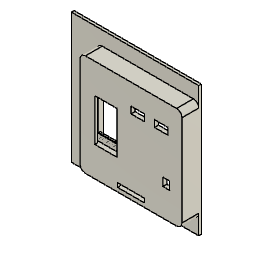
electronics_holder (Autodesk Fusion 360 design; units mm, degrees)
Autodesk Fusion 360 part; units mm, degrees
note: some values were not read from the file. Set by a fixed rule: which sketch regions a step uses.
sketch "Sketch1" plane through (0, 0, 0) normal (0, 1, 0) x (1, 0, 0)
  line L0 (0, 0) -> (190, 0)
  line L1 (190, 0) -> (190, -194)
  line L2 (190, -194) -> (0, -194)
  line L3 (0, -194) -> (0, 0)
  dimension "d1" = 190
  dimension "d2" = 194
  constraint horizontal L0
  constraint vertical L1
  constraint horizontal L2
  constraint vertical L3
  constraint coincident L0.start L3.end
  measures "d1" distance of L0.start L0.end
  measures "d2" distance of L0.end L1.end
extrude "Extrude1" add sketch "Sketch1" against normal blind 4
sketch "Sketch2" plane through (0, -4, 0) normal (0, -1, 0) x (1, 0, 0)
  line L0 (190, 194) -> (0, 194)
  line L1 (0, 194) -> (0, 0)
  line L2 (0, 0) -> (190, 0)
  line L3 (190, 0) -> (190, 194)
  line L4 (44, 167) -> (184, 167)
  line L5 (184, 167) -> (184, 27)
  line L6 (184, 27) -> (44, 27)
  line L7 (44, 27) -> (44, 167)
  dimension "d5" = 44
  dimension "d6" = 140
  dimension "d7" = 27
  dimension "d8" = 140
  constraint horizontal L4
  constraint vertical L5
  constraint horizontal L6
  constraint vertical L7
  measures "d5" distance of L1 L7
  measures "d6" distance of L5.end L6.end
  measures "d7" distance of L2 L6
  measures "d8" distance of L4.end L5.end
extrude "Extrude2" cut sketch "Sketch2" against normal blind 4 contours L4 L5 L6 L7
fillet "Fillet1" radius 8 4 edges at (44, -2, 167) (44, -2, 27) (184, -2, 167) (184, -2, 27)
sketch "Sketch3" plane through (0, -4, 0) normal (0, -1, 0) x (1, 0, 0)
  line L0 (184, 159) -> (184, 35)
  arc A0 (176, 27) -> (184, 35) centre (176, 35) ccw
  line L1 (176, 27) -> (52, 27)
  arc A1 (44, 35) -> (52, 27) centre (52, 35) ccw
  line L2 (44, 35) -> (44, 159)
  arc A2 (52, 167) -> (44, 159) centre (52, 159) ccw
  line L3 (52, 167) -> (176, 167)
  arc A3 (184, 159) -> (176, 167) centre (176, 159) ccw
  line L4 (190, 194) -> (0, 194)
  line L5 (0, 194) -> (0, 0)
  line L6 (0, 0) -> (190, 0)
  line L7 (190, 0) -> (190, 194)
  line L8 (38, 173) -> (190, 173)
  line L9 (190, 173) -> (190, 21)
  line L10 (190, 21) -> (38, 21)
  line L11 (38, 21) -> (38, 173)
  dimension "d13" = 6
  dimension "d14" = 6
  dimension "d15" = 6
  dimension "d16" = 6
  constraint horizontal L8
  constraint vertical L9
  constraint horizontal L10
  constraint vertical L11
  constraint coincident L7 L9.end
  measures "d13" distance of L0 L9
  measures "d14" distance of L2 L11
  measures "d15" distance of L1 L10
  measures "d16" distance of L3 L8
extrude "Extrude3" add sketch "Sketch3" along normal blind 21 contours L7 L8 L9 L10 L11
sketch "Sketch4" plane through (0, -25, 0) normal (0, -1, 0) x (1, 0, 0)
  arc A0 (176, 27) -> (184, 35) centre (176, 35) ccw
  line L0 (176, 27) -> (52, 27)
  arc A1 (44, 35) -> (52, 27) centre (52, 35) ccw
  line L1 (44, 35) -> (44, 159)
  arc A2 (52, 167) -> (44, 159) centre (52, 159) ccw
  line L2 (52, 167) -> (176, 167)
  arc A3 (184, 159) -> (176, 167) centre (176, 159) ccw
  line L3 (184, 159) -> (184, 35)
  line L4 (38, 21) -> (190, 21)
  line L5 (190, 21) -> (190, 173)
  line L6 (190, 173) -> (38, 173)
  line L7 (38, 173) -> (38, 21)
  line L8 (38, 173) -> (190, 173)
  line L9 (190, 173) -> (190, 21)
  line L10 (190, 21) -> (38, 21)
  line L11 (38, 21) -> (38, 173)
  constraint horizontal L8
  constraint vertical L9
  constraint horizontal L10
  constraint vertical L11
  constraint coincident L4.end L5.start
  constraint coincident L6.end L7.start
extrude "Extrude4" add sketch "Sketch4" along normal blind 4 contours A0 L0 A1 L1 A2 L2 A3 L3 | L4 L5 L6 L7 L8 L9 L10 L11
fillet "Fillet2" radius 8 4 edges at (38, -16.5, 173) (190, -16.5, 173) (38, -16.5, 21) (190, -16.5, 21)
sketch "Sketch5" plane through (0, 0, 0) normal (0, 1, 0) x (-1, 0, 0)
  line L0 (-184, 35) -> (-184, 159)
  arc A0 (-176, 167) -> (-184, 159) centre (-176, 159) ccw
  line L1 (-176, 167) -> (-52, 167)
  arc A1 (-44, 159) -> (-52, 167) centre (-52, 159) ccw
  line L2 (-44, 159) -> (-44, 35)
  arc A2 (-52, 27) -> (-44, 35) centre (-52, 35) ccw
  line L3 (-52, 27) -> (-176, 27)
  arc A3 (-184, 35) -> (-176, 27) centre (-176, 35) ccw
  line L4 (0, 194) -> (-190, 194)
  line L5 (-190, 194) -> (-190, 0)
  line L6 (-190, 0) -> (0, 0)
  line L7 (0, 0) -> (0, 194)
  line L8 (-64, 167) -> (-44, 167)
  line L9 (-44, 167) -> (-44, 147)
  line L10 (-44, 147) -> (-64, 147)
  line L11 (-64, 147) -> (-64, 167)
  circle A4 centre (-54, 157) radius 2.75
  line L12 (-164, 167) -> (-184, 167)
  line L13 (-184, 167) -> (-184, 147)
  line L14 (-184, 147) -> (-164, 147)
  line L15 (-164, 147) -> (-164, 167)
  line L16 (-184, 47) -> (-164, 47)
  line L17 (-164, 47) -> (-164, 27)
  line L18 (-164, 27) -> (-184, 27)
  line L19 (-184, 27) -> (-184, 47)
  line L20 (-44, 47) -> (-64, 47)
  line L21 (-64, 47) -> (-64, 27)
  line L22 (-64, 27) -> (-44, 27)
  line L23 (-44, 27) -> (-44, 47)
  circle A5 centre (-174, 157) radius 2.75
  circle A6 centre (-174, 37) radius 2.75
  circle A7 centre (-54, 37) radius 2.75
  dimension "d23" = 5.5
  dimension "d24" = 10
  dimension "d25" = 10
  dimension "d26" = 10
  dimension "d27" = 10
  dimension "d28" = 5.5
  dimension "d29" = 10
  dimension "d30" = 10
  dimension "d31" = 10
  dimension "d32" = 10
  dimension "d33" = 5.5
  dimension "d34" = 5.5
  dimension "d35" = 10
  dimension "d36" = 10
  dimension "d37" = 10
  dimension "d38" = 10
  dimension "d39" = 10
  dimension "d40" = 10
  dimension "d41" = 10
  dimension "d42" = 10
  constraint horizontal L8
  constraint vertical L9
  constraint horizontal L10
  constraint vertical L11
  constraint coincident L2 L9.end
  constraint coincident L1 L8.start
  constraint horizontal L12
  constraint vertical L13
  constraint horizontal L14
  constraint vertical L15
  constraint coincident L0 L13.end
  constraint coincident L1 L12.start
  constraint horizontal L16
  constraint vertical L17
  constraint horizontal L18
  constraint vertical L19
  constraint coincident L3 L17.end
  constraint coincident L0 L16.start
  constraint horizontal L20
  constraint vertical L21
  constraint horizontal L22
  constraint vertical L23
  constraint coincident L3 L21.end
  constraint coincident L2 L20.start
  measures "d23" diameter of A4
  measures "d24" distance of L9 A4.centre
  measures "d25" distance of L8 A4.centre
  measures "d26" distance of L11 A4.centre
  measures "d27" distance of L10 A4.centre
  measures "d28" diameter of A5
  measures "d29" distance of L12 A5.centre
  measures "d30" distance of L13 A5.centre
  measures "d31" distance of L15 A5.centre
  measures "d32" distance of L14 A5.centre
  measures "d33" diameter of A6
  measures "d34" diameter of A7
  measures "d35" distance of L23 A7.centre
  measures "d36" distance of L22 A7.centre
  measures "d37" distance of L20 A7.centre
  measures "d38" distance of L21 A7.centre
  measures "d39" distance of L17 A6.centre
  measures "d40" distance of L19 A6.centre
  measures "d41" distance of L18 A6.centre
  measures "d42" distance of L16 A6.centre
extrude "Extrude5" add sketch "Sketch5" against normal blind 6 contours L0 L3 A3 L16 L17 L18 L19 | A3 L18 L19 | L0 A0 L1 L12 L13 L14 L15 | A0 L12 L13 | L2 A2 L3 L20 L21 L22 L23 | A2 L22 L23 | L1 A1 L2 L8 L9 L10 L11 | A1 L8 L9 | A4 | A5 | A6 | A7
extrude "Extrude6" cut sketch "Sketch5" against normal blind 1.5 contours A4 | A5 | A6 | A7
fillet "Fillet3" radius 8 4 edges at (164, -3, 147) (164, -3, 47) (64, -3, 47) (64, -3, 147)
sketch "Sketch6" plane through (0, -25, 0) normal (0, 1, 0) x (-1, 0, 0)
  arc A0 (-52, 27) -> (-44, 35) centre (-52, 35) ccw
  line L0 (-44, 35) -> (-44, 159)
  arc A1 (-44, 159) -> (-52, 167) centre (-52, 159) ccw
  line L1 (-52, 167) -> (-176, 167)
  arc A2 (-176, 167) -> (-184, 159) centre (-176, 159) ccw
  line L2 (-184, 159) -> (-184, 35)
  arc A3 (-184, 35) -> (-176, 27) centre (-176, 35) ccw
  line L3 (-176, 27) -> (-52, 27)
  line L4 (-93, 128.5) -> (-60, 128.5)
  line L5 (-60, 128.5) -> (-60, 65.5)
  line L6 (-60, 65.5) -> (-93, 65.5)
  line L7 (-93, 65.5) -> (-93, 128.5)
  dimension "d51" = 63
  dimension "d54" = 33
  dimension "d88" = 16
  dimension "d92" = 38.5
  constraint horizontal L4
  constraint vertical L5
  constraint horizontal L6
  constraint vertical L7
  measures "d51" distance of L4.end L5.end
  measures "d54" distance of L4.start L4.end
  measures "d88" distance of L0 L5
  measures "d92" distance of L1 L4
extrude "Extrude7" cut sketch "Sketch6" against normal blind 4 contours L4 L5 L6 L7
sketch "Sketch7" plane through (0, -25, 0) normal (0, 1, 0) x (-1, 0, 0)
  line L0 (-60, 128.5) -> (-60, 65.5)
  line L1 (-60, 65.5) -> (-93, 65.5)
  line L2 (-93, 65.5) -> (-93, 128.5)
  line L3 (-93, 128.5) -> (-60, 128.5)
  arc A0 (-52, 27) -> (-44, 35) centre (-52, 35) ccw
  line L4 (-44, 35) -> (-44, 159)
  arc A1 (-44, 159) -> (-52, 167) centre (-52, 159) ccw
  line L5 (-52, 167) -> (-176, 167)
  arc A2 (-176, 167) -> (-184, 159) centre (-176, 159) ccw
  line L6 (-184, 159) -> (-184, 35)
  arc A3 (-184, 35) -> (-176, 27) centre (-176, 35) ccw
  line L7 (-176, 27) -> (-52, 27)
  line L8 (-96, 130.6162) -> (-99, 130.6162)
  line L9 (-99, 130.6162) -> (-99, 62.5)
  line L10 (-99, 62.5) -> (-96, 62.5)
  line L11 (-96, 62.5) -> (-96, 130.6162)
  line L12 (-96, 62.5) -> (-54, 62.5)
  line L13 (-54, 62.5) -> (-54, 65.5)
  line L14 (-54, 65.5) -> (-96, 65.5)
  line L15 (-96, 65.5) -> (-96, 62.5)
  line L16 (-54, 65.5) -> (-57, 65.5)
  line L17 (-57, 65.5) -> (-57, 130.6162)
  line L18 (-57, 130.6162) -> (-54, 130.6162)
  line L19 (-54, 130.6162) -> (-54, 65.5)
  dimension "d55" = 3
  dimension "d56" = 3
  dimension "d57" = 3
  dimension "d58" = 3
  dimension "d59" = 3
  constraint horizontal L8
  constraint vertical L9
  constraint horizontal L10
  constraint vertical L11
  constraint horizontal L12
  constraint vertical L13
  constraint horizontal L14
  constraint vertical L15
  constraint horizontal L16
  constraint vertical L17
  constraint horizontal L18
  constraint vertical L19
  constraint collinear L1 L14
  measures "d55" distance of L2 L11
  measures "d56" distance of L0 L17
  measures "d57" distance of L8.start L8.end
  measures "d58" distance of L17.end L18.end
  measures "d59" distance of L12.end L13.end
extrude "Extrude8" add sketch "Sketch7" along normal blind 4 contours L1 L11 L12 L13 L14 L15 L16 | L14 L16 L17 L18 L19 | L8 L9 L10 L11 L15
sketch "Sketch8" plane through (0, -25, 0) normal (0, 1, 0) x (-1, 0, 0)
  line L0 (-96, 65.5) -> (-93, 65.5)
  line L1 (-93, 65.5) -> (-93, 128.5)
  line L2 (-93, 128.5) -> (-60, 128.5)
  line L3 (-60, 128.5) -> (-60, 65.5)
  line L4 (-60, 65.5) -> (-57, 65.5)
  line L5 (-57, 65.5) -> (-57, 130.6162)
  line L6 (-57, 130.6162) -> (-54, 130.6162)
  line L7 (-54, 130.6162) -> (-54, 62.5)
  line L8 (-54, 62.5) -> (-99, 62.5)
  line L9 (-99, 62.5) -> (-99, 130.6162)
  line L10 (-99, 130.6162) -> (-96, 130.6162)
  line L11 (-96, 130.6162) -> (-96, 65.5)
  arc A0 (-52, 27) -> (-44, 35) centre (-52, 35) ccw
  line L12 (-44, 35) -> (-44, 159)
  arc A1 (-44, 159) -> (-52, 167) centre (-52, 159) ccw
  line L13 (-52, 167) -> (-176, 167)
  arc A2 (-176, 167) -> (-184, 159) centre (-176, 159) ccw
  line L14 (-184, 159) -> (-184, 35)
  arc A3 (-184, 35) -> (-176, 27) centre (-176, 35) ccw
  line L15 (-176, 27) -> (-52, 27)
  line L16 (-174, 142) -> (-144, 142)
  line L17 (-144, 142) -> (-144, 89)
  line L18 (-144, 89) -> (-174, 89)
  line L19 (-174, 89) -> (-174, 142)
  line L20 (-109, 142) -> (-139, 142)
  line L21 (-139, 142) -> (-139, 89)
  line L22 (-139, 89) -> (-109, 89)
  line L23 (-109, 89) -> (-109, 142)
  line L24 (-171.5, 84) -> (-111.5, 84)
  line L25 (-111.5, 84) -> (-111.5, 52)
  line L26 (-111.5, 52) -> (-171.5, 52)
  line L27 (-171.5, 52) -> (-171.5, 84)
  dimension "d60" = 30
  dimension "d61" = 53
  dimension "d64" = 30
  dimension "d65" = 53
  dimension "d66" = 60
  dimension "d67" = 32
  dimension "d86" = 5
  dimension "d87" = 25
  dimension "d89" = 10
  dimension "d90" = 5
  dimension "d91" = 2.5
  constraint horizontal L16
  constraint vertical L17
  constraint horizontal L18
  constraint vertical L19
  constraint horizontal L20
  constraint vertical L21
  constraint horizontal L22
  constraint vertical L23
  constraint horizontal L24
  constraint vertical L25
  constraint horizontal L26
  constraint vertical L27
  constraint collinear L16 L20
  measures "d60" distance of L16.start L16.end
  measures "d61" distance of L16.end L17.end
  measures "d64" distance of L20.start L20.end
  measures "d65" distance of L20.start L22.end
  measures "d66" distance of L24.start L24.end
  measures "d67" distance of L24.start L26.end
  measures "d86" distance of L22 L24
  measures "d87" distance of L13 L16
  measures "d89" distance of L9 L23
  measures "d90" distance of L17 L21
  measures "d91" distance of L19 L27
extrude "Extrude9" add sketch "Sketch8" along normal blind 2 contours L16 L17 L18 L19 | L20 L21 L22 L23 | L24 L25 L26 L27
sketch "Sketch9" plane through (0, -25, 0) normal (0, 1, 0) x (-1, 0, 0)
  line L0 (-171.5, 52) -> (-171.5, 84)
  line L1 (-171.5, 84) -> (-111.5, 84)
  line L2 (-111.5, 84) -> (-111.5, 52)
  line L3 (-111.5, 52) -> (-171.5, 52)
  line L4 (-109, 89) -> (-139, 89)
  line L5 (-139, 89) -> (-139, 142)
  line L6 (-139, 142) -> (-109, 142)
  line L7 (-109, 142) -> (-109, 89)
  line L8 (-174, 89) -> (-174, 142)
  line L9 (-174, 142) -> (-144, 142)
  line L10 (-144, 142) -> (-144, 89)
  line L11 (-144, 89) -> (-174, 89)
  line L12 (-96, 65.5) -> (-93, 65.5)
  line L13 (-93, 65.5) -> (-93, 128.5)
  line L14 (-93, 128.5) -> (-60, 128.5)
  line L15 (-60, 128.5) -> (-60, 65.5)
  line L16 (-60, 65.5) -> (-57, 65.5)
  line L17 (-57, 65.5) -> (-57, 130.6162)
  line L18 (-57, 130.6162) -> (-54, 130.6162)
  line L19 (-54, 130.6162) -> (-54, 62.5)
  line L20 (-54, 62.5) -> (-99, 62.5)
  line L21 (-99, 62.5) -> (-99, 130.6162)
  line L22 (-99, 130.6162) -> (-96, 130.6162)
  line L23 (-96, 130.6162) -> (-96, 65.5)
  arc A0 (-52, 27) -> (-44, 35) centre (-52, 35) ccw
  line L24 (-44, 35) -> (-44, 159)
  arc A1 (-44, 159) -> (-52, 167) centre (-52, 159) ccw
  line L25 (-52, 167) -> (-176, 167)
  arc A2 (-176, 167) -> (-184, 159) centre (-176, 159) ccw
  line L26 (-184, 159) -> (-184, 35)
  arc A3 (-184, 35) -> (-176, 27) centre (-176, 35) ccw
  line L27 (-176, 27) -> (-52, 27)
  line L28 (-134, 27) -> (-94, 27)
  line L29 (-94, 27) -> (-94, 33)
  line L30 (-94, 33) -> (-134, 33)
  line L31 (-134, 33) -> (-134, 27)
  dimension "d68" = 6
  dimension "d70" = 50
  dimension "d71" = 50
  dimension "d103" = 40
  constraint horizontal L28
  constraint vertical L29
  constraint horizontal L30
  constraint vertical L31
  constraint coincident L27 L28.start
  measures "d68" distance of L28.start L30.end
  measures "d70" distance of L26 L31
  measures "d71" distance of L24 L29
  measures "d103" distance of L29.end L30.end
extrude "Extrude10" cut sketch "Sketch9" against normal blind 4 contours L27 L28 L29 L30 L31
sketch "Sketch10" plane through (0, -25, 0) normal (0, 1, 0) x (-1, 0, 0)
  line L0 (-134, 27) -> (-134, 33)
  line L1 (-134, 33) -> (-94, 33)
  line L2 (-94, 33) -> (-94, 27)
  line L3 (-94, 27) -> (-52, 27)
  arc A0 (-52, 27) -> (-44, 35) centre (-52, 35) ccw
  line L4 (-44, 35) -> (-44, 159)
  arc A1 (-44, 159) -> (-52, 167) centre (-52, 159) ccw
  line L5 (-52, 167) -> (-176, 167)
  arc A2 (-176, 167) -> (-184, 159) centre (-176, 159) ccw
  line L6 (-184, 159) -> (-184, 35)
  arc A3 (-184, 35) -> (-176, 27) centre (-176, 35) ccw
  line L7 (-176, 27) -> (-134, 27)
  line L8 (-96, 65.5) -> (-93, 65.5)
  line L9 (-93, 65.5) -> (-93, 128.5)
  line L10 (-93, 128.5) -> (-60, 128.5)
  line L11 (-60, 128.5) -> (-60, 65.5)
  line L12 (-60, 65.5) -> (-57, 65.5)
  line L13 (-57, 65.5) -> (-57, 130.6162)
  line L14 (-57, 130.6162) -> (-54, 130.6162)
  line L15 (-54, 130.6162) -> (-54, 62.5)
  line L16 (-54, 62.5) -> (-99, 62.5)
  line L17 (-99, 62.5) -> (-99, 130.6162)
  line L18 (-99, 130.6162) -> (-96, 130.6162)
  line L19 (-96, 130.6162) -> (-96, 65.5)
  line L20 (-174, 89) -> (-174, 142)
  line L21 (-174, 142) -> (-144, 142)
  line L22 (-144, 142) -> (-144, 89)
  line L23 (-144, 89) -> (-174, 89)
  line L24 (-109, 89) -> (-139, 89)
  line L25 (-139, 89) -> (-139, 142)
  line L26 (-139, 142) -> (-109, 142)
  line L27 (-109, 142) -> (-109, 89)
  line L28 (-171.5, 52) -> (-171.5, 84)
  line L29 (-171.5, 84) -> (-111.5, 84)
  line L30 (-111.5, 84) -> (-111.5, 52)
  line L31 (-111.5, 52) -> (-171.5, 52)
  line L32 (-184, 37) -> (-44, 37)
  line L33 (-44, 37) -> (-44, 33)
  line L34 (-44, 33) -> (-184, 33)
  line L35 (-184, 33) -> (-184, 37)
  dimension "d74" = 4
  constraint horizontal L32
  constraint vertical L33
  constraint horizontal L34
  constraint vertical L35
  constraint collinear L1 L34
  constraint collinear L4 L33
  constraint collinear L6 L35
  measures "d74" distance of L32 L34
extrude "Extrude11" add sketch "Sketch10" along normal blind 19 contours L1 A0 L4 L6 A3 L32 L33 L34 L35 | A3 L34 L35 | A0 L33 L34
sketch "Sketch11" plane through (0, -23, 0) normal (0, 1, 0) x (-1, 0, 0)
  line L0 (-174, 89) -> (-144, 89)
  line L1 (-144, 89) -> (-144, 142)
  line L2 (-144, 142) -> (-174, 142)
  line L3 (-174, 142) -> (-174, 89)
  line L4 (-169, 142) -> (-149, 142)
  line L5 (-149, 142) -> (-149, 132)
  line L6 (-149, 132) -> (-169, 132)
  line L7 (-169, 132) -> (-169, 142)
  line L8 (-134, 132) -> (-114, 132)
  line L9 (-114, 132) -> (-114, 142)
  line L10 (-114, 142) -> (-134, 142)
  line L11 (-134, 142) -> (-134, 132)
  line L12 (-171.5, 74) -> (-161.5, 74)
  line L13 (-161.5, 74) -> (-161.5, 62)
  line L14 (-161.5, 62) -> (-171.5, 62)
  line L15 (-171.5, 62) -> (-171.5, 74)
  line L16 (-171.5, 84) -> (-171.5, 52)
  line L17 (-111.5, 84) -> (-171.5, 84)
  line L18 (-171.5, 52) -> (-111.5, 52)
  line L19 (-111.5, 52) -> (-111.5, 84)
  line L20 (-111.5, 84) -> (-171.5, 84)
  line L21 (-171.5, 84) -> (-171.5, 52)
  line L22 (-109, 142) -> (-139, 142)
  line L23 (-109, 89) -> (-109, 142)
  line L24 (-139, 142) -> (-139, 89)
  dimension "d93" = 10
  dimension "d94" = 10
  dimension "d95" = 10
  dimension "d96" = 5
  dimension "d97" = 5
  dimension "d98" = 10
  dimension "d100" = 10
  dimension "d101" = 5
  dimension "d102" = 5
  constraint horizontal L4
  constraint vertical L5
  constraint horizontal L6
  constraint vertical L7
  constraint horizontal L8
  constraint vertical L9
  constraint horizontal L10
  constraint vertical L11
  constraint horizontal L12
  constraint vertical L13
  constraint horizontal L14
  constraint vertical L15
  constraint collinear L15 L16
  constraint collinear L4 L10
  constraint collinear L2 L4
  measures "d93" distance of L12.start L12.end
  measures "d94" distance of L12 L17
  measures "d95" distance of L14 L18
  measures "d96" distance of L1 L5
  measures "d97" distance of L3 L7
  measures "d98" distance of L4.end L5.end
  measures "d100" distance of L8 L22
  measures "d101" distance of L9 L23
  measures "d102" distance of L11 L24
extrude "Extrude12" cut sketch "Sketch11" against normal blind 6 contours L2 L4 L5 L6 L7 | L8 L9 L10 L11 L22 | L12 L13 L14 L15 L16 L21
sketch "Sketch12" plane through (0, -21, 0) normal (0, 1, 0) x (-1, 0, 0)
  line L0 (-57, 65.5) -> (-96, 65.5)
  line L1 (-96, 65.5) -> (-96, 130.6162)
  line L2 (-96, 130.6162) -> (-99, 130.6162)
  line L3 (-99, 130.6162) -> (-99, 62.5)
  line L4 (-99, 62.5) -> (-54, 62.5)
  line L5 (-54, 62.5) -> (-54, 130.6162)
  line L6 (-54, 130.6162) -> (-57, 130.6162)
  line L7 (-57, 130.6162) -> (-57, 65.5)
  line L8 (-99, 62.5) -> (-54, 62.5)
  line L9 (-54, 62.5) -> (-54, 75.5)
  line L10 (-54, 75.5) -> (-99, 75.5)
  line L11 (-99, 75.5) -> (-99, 62.5)
  dimension "d79" = 10
  constraint horizontal L8
  constraint vertical L9
  constraint horizontal L10
  constraint vertical L11
  constraint coincident L5 L9.end
  constraint coincident L3.end L4.start
  measures "d79" distance of L0 L10
extrude "Extrude13" add sketch "Sketch12" against normal blind 1 contours L0 L1 L3 L4 L5 L7 L8 L9 L10 L11 | L0 L1 L7 L10
sketch "Sketch13" plane through (0, -21, 0) normal (0, 1, 0) x (-1, 0, 0)
  line L0 (-54, 62.5) -> (-54, 130.6162)
  line L1 (-54, 130.6162) -> (-57, 130.6162)
  line L2 (-57, 130.6162) -> (-57, 75.5)
  line L3 (-57, 75.5) -> (-96, 75.5)
  line L4 (-96, 75.5) -> (-96, 130.6162)
  line L5 (-96, 130.6162) -> (-99, 130.6162)
  line L6 (-99, 130.6162) -> (-99, 62.5)
  line L7 (-99, 62.5) -> (-54, 62.5)
  line L8 (-99, 72) -> (-54, 72)
  line L9 (-54, 72) -> (-54, 70)
  line L10 (-54, 70) -> (-99, 70)
  line L11 (-99, 70) -> (-99, 72)
  dimension "d82" = 2
  constraint horizontal L8
  constraint vertical L9
  constraint horizontal L10
  constraint vertical L11
  constraint coincident L0 L9.end
  constraint coincident L6 L8.start
  measures "d82" distance of L8.end L9.end
extrude "Extrude14" add sketch "Sketch13" along normal blind 6 contours L0 L6 L8 L9 L10 L11
equation "d1 = 184 mm + ( ( 12 / 2 ) * 1 mm )"
equation "d2 = 140 mm + ( ( 2 * 27 ) * 1 mm )"
equation "d24 = 7.25 mm + ( ( 5.5 / 2 ) * 1 mm )"
equation "d25 = 7.25 mm + ( ( 5.5 / 2 ) * 1 mm )"
equation "d55 = ( ( 39 - 33 ) / 2 ) * 1 mm"
equation "d56 = ( ( 39 - 33 ) / 2 ) * 1 mm"
named bodies: "Electronics Holder"
